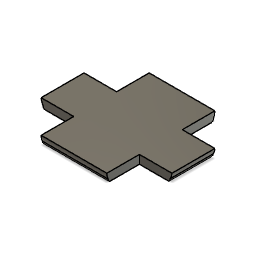
CUBE2025年5月31日 (Autodesk Fusion 360 design; units mm, degrees)
Autodesk Fusion 360 part; units mm, degrees
sketch "草图1" plane through (0, 0, 0) normal (0, 1, 0) x (1, 0, 0)
  line L0 (11.6, 19.075, 3) -> (-11.6, 19.075, 3)
  line L1 (-23.1, 7.575, 3) -> (-23.1, -7.575, 3)
  line L2 (-11.6, -19.075, 3) -> (11.6, -19.075, 3)
  line L3 (23.1, -7.575, 3) -> (23.1, 7.575, 3)
  arc A0 through (-11.6, 19.075, 3) (-19.7317, 15.7067, 3) (-23.1, 7.575, 3)
  arc A1 through (23.1, 7.575, 3) (19.7317, 15.7067, 3) (11.6, 19.075, 3)
  arc A2 through (11.6, -19.075, 3) (19.7317, -15.7067, 3) (23.1, -7.575, 3)
  arc A3 through (-23.1, -7.575, 3) (-19.7317, -15.7067, 3) (-11.6, -19.075, 3)
  point P0 (23.1, 19.075)
  point P1 (-23.1, 19.075)
  point P2 (23.1, -19.075)
  dimension "d5" = 46.2
  dimension "d6" = 38.15
  dimension "d16" = 11.5
  dimension "d17" = 11.5
  dimension "d18" = 11.5
  dimension "d19" = 11.5
  measures "d5" distance of P0 P1
  measures "d6" distance of P0 P2
sketch "草图2" plane through (0, 0, 0) normal (0, 1, 0) x (1, 0, 0)
  circle A0 centre (17.3934, 13.5745) radius 0.65
  circle A1 centre (-17.3935, -13.5745) radius 0.65
  circle A2 centre (17.3934, -13.5745) radius 0.65
  circle A3 centre (-17.3935, 13.5745) radius 0.65
  line L0 (16.0995, 15.5745) -> (-16.0995, 15.5745)
  line L1 (-16.0995, -15.5745) -> (16.0995, -15.5745)
  line L2 (-19.3935, 12.4745) -> (-19.3935, -12.4745)
  arc A4 (-19.3935, -12.4745) -> (-16.0995, -15.5745) centre (-16.0995, -12.2745) ccw
  arc A5 (19.3934, 12.4745) -> (16.0995, 15.5745) centre (16.0995, 12.2745) ccw
  arc A6 (16.0995, -15.5745) -> (19.3934, -12.4745) centre (16.0995, -12.2745) ccw
  line L3 (19.3934, -12.4745) -> (19.3934, 12.4745)
  arc A7 (-16.0995, 15.5745) -> (-19.3935, 12.4745) centre (-16.0995, 12.2745) ccw
  line L4 (-17.3935, 13.5745) -> (17.3934, -13.5745)
  line L5 (17.3934, 13.5745) -> (-17.3935, -13.5745)
  constraint coincident A3.centre L4.start
  constraint coincident A2.centre L4.end
  constraint coincident A0.centre L5.start
  constraint coincident A1.centre L5.end
sketch "草图3" plane through (0, 0, 0) normal (0, 1, 0) x (1, 0, 0)
  line L0 (21.945, 18.1212) -> (-21.945, 18.1212)
  line L1 (-21.945, 18.1212) -> (-21.945, -18.1213)
  line L2 (-21.945, -18.1213) -> (21.945, -18.1213)
  line L3 (21.945, -18.1213) -> (21.945, 18.1212)
  circle A0 centre (11.02, -7.1963) radius 10.925
  circle A1 centre (11.02, 7.1962) radius 10.925
  circle A2 centre (-11.02, 7.1962) radius 10.925
  circle A3 centre (-11.02, -7.1963) radius 10.925
sketch "草图4" plane through (0, 0, 0) normal (1, 0, 0) x (0, 0, -1)
  line L0 (18.1213, 0.0001) -> (-18.1217, 0.0001)
  line L1 (-18.1217, 0.0001) -> (-18.1217, 1.0001)
  line L2 (-18.1217, 1.0001) -> (18.1213, 1.0001)
  line L3 (18.1213, 1.0001) -> (18.1213, 0.0001)
  line L4 (-18.1217, 1.0001) -> (-18.6217, 1.0001)
  circle A0 centre (-17.3717, 1.0001) radius 1.25
  line L5 (18.1213, 1.0001) -> (18.6213, 1.0001)
  line L6 (19.5, 0) -> (19.2829, 0)
  line L7 (18.1212, 0) -> (-18.1213, 0)
  circle A1 centre (17.3713, 1.0001) radius 1.25
  line L8 (19.075, 3) -> (-19.075, 3)
  circle A2 centre (14.3251, 3.0262) radius 4.75
  circle A3 centre (-14.3251, 3.0254) radius 4.75
  dimension "d7" = 36.243
  dimension "d8" = 1
  dimension "d9" = 0.5
  dimension "d10" = 2.5
  dimension "d12" = 0.5
  dimension "d13" = 2.5
  dimension "d20" = 9.5
  dimension "d21" = 9.5
  constraint horizontal L0
  constraint vertical L1
  constraint horizontal L2
  constraint vertical L3
  constraint perpendicular L1 L4
  constraint coincident L0.end A0
  constraint coincident L4.end A0
  constraint perpendicular L3 L5
  constraint horizontal L6
  constraint collinear L6 L7
  constraint coincident L5.end A1
  constraint coincident L7.start A1
  constraint horizontal L8
  constraint coincident L8.start A2
  constraint coincident L5.end A2
  constraint coincident L8.end A3
  constraint coincident L4.end A3
  measures "d7" distance of L0.start L0.end
  measures "d8" distance of L0.end L1.end
  measures "d9" distance of L1.end L4.end
  measures "d10" diameter of A0
  measures "d12" distance of L2.end L5.end
  measures "d13" diameter of A1
  measures "d20" diameter of A2
  measures "d21" diameter of A3
extrude "拉伸1" add sketch "草图4" along normal blind 11.6 contours L0 L3 L7 A2 | L3 A1 A2 | L0 L2 L3 L7 A1 A2 | L3 L5 A2 | L2 L5 A1 | L2 A1 L8 A2 | L0 L2 L7 A1 A2 | L0 L2 L7 A2 A3 | L2 L8 A2 A3 | L0 L2 A0 L7 A3 | L2 A0 L8 A3 | L0 L1 L2 A0 L7 A3 | L2 L4 A0 | L0 L1 L7 A3 | L1 A0 A3 | L1 L4 A3 makes body 1
extrude "拉伸2" add 1 faces at (0, 1.0001, -3.1919) along direction (-1, 0, 0) blind 11.6 on bodies 1 bodies 1
sketch "草图5" plane through (0, 0, 0) normal (0, 0, 1) x (1, 0, 0)
  line L0 (-21.945, 0) -> (21.945, 0)
  line L1 (21.945, 0) -> (21.945, 1)
  line L2 (21.945, 1) -> (-21.945, 1)
  line L3 (-21.945, 1) -> (-21.945, 0)
  line L4 (21.945, 1) -> (22.445, 1)
  circle A0 centre (21.195, 1) radius 1.25
  circle A1 centre (18.3706, 3.4416) radius 4.75
  line L5 (-21.945, 1) -> (-22.445, 1)
  circle A2 centre (-21.195, 1) radius 1.25
  circle A3 centre (-18.3706, 3.4416) radius 4.75
  line L6 (-23.1, 3) -> (23.1, 3)
  dimension "d26" = 43.89
  dimension "d27" = 1
  dimension "d28" = 0.5
  dimension "d29" = 2.5
  dimension "d30" = 9.5
  dimension "d31" = 0.5
  dimension "d32" = 2.5
  dimension "d33" = 9.5
  constraint horizontal L0
  constraint vertical L1
  constraint horizontal L2
  constraint vertical L3
  constraint perpendicular L1 L4
  constraint coincident L4.end A0
  constraint coincident L0.end A0
  constraint coincident L4.end A1
  constraint perpendicular L3 L5
  constraint coincident L5.end A2
  constraint coincident L0.start A2
  constraint coincident L5.end A3
  constraint coincident A3 L6.start
  constraint coincident A1 L6.end
  constraint horizontal L6
  measures "d26" distance of L0.start L0.end
  measures "d27" distance of L0.end L1.end
  measures "d28" distance of L1.end L4.end
  measures "d29" diameter of A0
  measures "d30" diameter of A1
  measures "d31" distance of L2.end L5.end
  measures "d32" diameter of A2
  measures "d33" diameter of A3
extrude "拉伸3" add sketch "草图5" along normal blind 1 separate body contours L0 L3 A3 | L3 A2 A3 | L0 L2 L3 A2 A3 | L3 L5 A3 | L2 L5 A2 | L2 A2 A3 L6 | L0 L2 A2 A3 | L0 L2 A1 A3 | L2 A1 A3 L6 | L0 L2 A0 A1 | L2 A0 A1 L6 | L0 L1 L2 A0 A1 | L2 L4 A0 | L0 L1 A1 | L1 A0 A1 | L1 L4 A1 makes body 2
extrude "拉伸4" add 1 faces at (4.5471, 1, 0) along direction (0, 0, -1) blind 7.575 on bodies 2 bodies 2
extrude "拉伸5" add 1 faces at (7.315, 2, 1) along direction (0, 0, 1) blind 6.575 on bodies 2 bodies 2
combine "合并1" operation add target body 2 tool bodies 1
